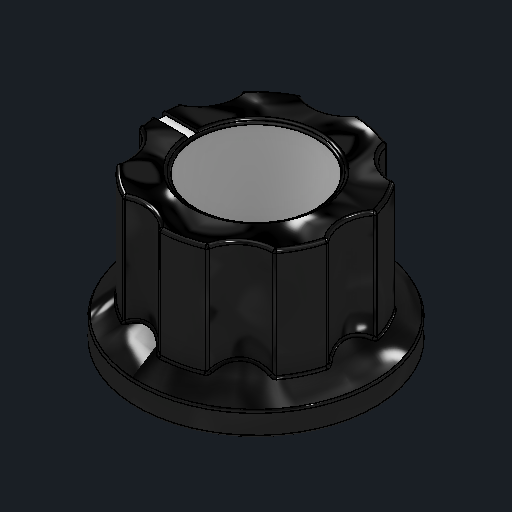
# Autodesk Inventor part: Knob2
Saved by Autodesk Inventor 2026.2 (Build 302298000, 298)
## iProperties
Created: 2015-05-06
Part Number: Knob2
Material: Generic
Document SubType Name: Modeling
Designer: Philip
Density: 1 g/cm^3
Appearance: Black
Author: Philip
Autodesk Inventor part; units mm, degrees
ref_plane "XZ Plane" through (0, 0, 0) normal (0, 1, 0) x (-1, 0, 0)
ref_plane "XY Plane" through (0, 0, 0) normal (0, 0, 1) x (1, 0, 0)
sketch "Sketch2" plane through (0, 0, 0) normal (0, 1, 0) x (-1, 0, 0)
  circle A0 centre (0, 0) radius 7.9375
  dimension "d0" = 15.875
  constraints: 1 centre point, 1 coincident
  measures "d0" diameter of A0
extrude "Extrusion1" add sketch "Sketch2" along normal blind 11.938
sketch "Sketch3" plane through (0, 11.938, 0) normal (0, 1, 0) x (1, 0, 0)
  circle A0 centre (0, 0) radius 7.9375 projected
  arc A1 (7.7055, 1.905) -> (7.7055, -1.905) centre (9.9648, 0) ccw
  line L0 (7.7055, -1.905) -> (7.7055, 1.905)
  dimension "d3" = 3.81
  constraints: 4 point on circle, 2 end point, 1 centre point, 1 vertical
  measures "d3" distance of L0.start L0.end
extrude "Extrusion2" cut sketch "Sketch3" against normal blind 11.938 contours A0 L0 | L0 A1
pattern_circular "Circular Pattern1" count 7 over 360 about axis through (0, 0, 0) along (0, 1, 0) of "Extrusion2"
sketch "Sketch4" plane through (0, 11.938, 0) normal (0, 1, 0) x (1, 0, 0)
  circle A0 centre (0, 0) radius 5.08
  dimension "d9" = 10.16
  constraints: 1 centre point, 1 coincident
  measures "d9" diameter of A0
extrude "Extrusion3" cut sketch "Sketch4" against normal blind 0.254
sketch "Sketch5" plane through (0, 0, 0) normal (1, 0, 0) x (0, 1, 0)
  line L0 (0, 0) -> (0, -9.525)
  line L1 (0, -9.525) -> (1.905, -9.525)
  line L2 (1.905, -9.525) -> (6.2153, -3.6691)
  line L3 (6.2153, -3.6691) -> (0, 0)
  line L4 (-2.3876, 0) -> (14.3256, 0) projected
  dimension "d12" = 9.525
  dimension "d13" = 1.905
  constraints: 8 end point, 1 perpendicular, 1 vertical
  measures "d12" distance of L0.start L0.end
  measures "d13" distance of L0.end L1.end
revolve "Revolution1" add sketch "Sketch5" angle 360 about axis through (0, -10, 0) along (0, 1, 0)
fillet "Fillet1" radius 0.254 31 edges at (0, 0, 9.525) (0, 1.905, 9.525) (-1.5598, 11.938, -6.8338) (0.1426, 7.5057, -7.9362) (-3.5719, 7.5057, -7.0884) (-6.1159, 7.5057, -5.0596) (-4.949, 11.938, -6.2058) (-6.3154, 11.938, -3.0413) (-7.769, 7.5057, -1.6269) (-7.769, 7.5057, 1.6269) (-7.9375, 11.938, 0) (-6.3154, 11.938, 3.0413) (-6.1159, 7.5057, 5.0596) (-3.5719, 7.5057, 7.0884) (-4.949, 11.938, 6.2058) (-1.5598, 11.938, 6.8338) (0.1426, 7.5057, 7.9362) (3.3149, 7.5057, 7.2122) (1.7663, 11.938, 7.7385) (4.3704, 11.938, 5.4803) (6.2937, 7.5057, 4.8367) (7.7055, 7.5057, 1.905) (7.1514, 11.938, 3.444) (7.0096, 11.938, 0) (7.7055, 7.5057, -1.905) (6.2937, 7.5057, -4.8367) (7.1514, 11.938, -3.444) (4.3704, 11.938, -5.4803) (3.3149, 7.5057, -7.2122) (1.7663, 11.938, -7.7385) (-5.08, 11.938, 0)
fillet "Fillet1" radius 0.254 16 edges at (-1.7312, 3.7511, -6.8) (-4.949, 3.0735, -6.2058) (-6.3154, 3.7565, -3.0414) (-7.9375, 3.0735, 0) (-6.3154, 3.7565, 3.0413) (-4.949, 3.0735, 6.2058) (-1.5598, 3.7565, 6.8338) (1.7663, 3.0735, 7.7385) (4.3703, 3.7565, 5.4803) (7.1514, 3.0735, 3.444) (7.0096, 3.7565, 0.0001) (7.1514, 3.0735, -3.444) (4.3704, 3.7565, -5.4802) (1.7663, 3.0735, -7.7385) (0.0738, 3.1388, -7.8484) (-5.08, 11.684, 0)
sketch "Sketch6" plane through (0, 11.938, 0) normal (0, 1, 0) x (1, 0, 0)
  circle A0 centre (0, 0) radius 5.046 projected
  line L0 (-5.0264, 0.4445) -> (-8.0286, 0.4445)
  line L1 (-8.0286, -0.4445) -> (-5.0264, -0.4445)
  arc A1 (-7.896, 1.5195) -> (-7.896, -1.5195) centre (0, 0) ccw projected
  dimension "d17" = 0.889
  dimension "d18" = 0.4445
  constraints: 4 end point, 4 point on circle, 2 horizontal
  measures "d17" distance between parallel lines of L1 L0
  measures "d18" distance from line of point (0, 0) L0
extrude "Extrusion4" cut sketch "Sketch6" against normal blind 0.254 contours A0 L1 A1 L0
ref_plane "Work Plane1" through (-7.9375, 0, 0) normal (1, 0, 0) x (0, 1, 0)
sketch "Sketch7" plane through (-7.9375, 0, 0) normal (1, 0, 0) x (0, 1, 0)
  line L0 (11.684, -0.4445) -> (11.684, 0.4445) projected
  line L1 (11.684, -0.4445) -> (3.2019, -0.4445)
  line L2 (3.2019, 1.5) -> (3.2019, -1.5) projected
  line L3 (11.684, 0.4445) -> (3.2019, 0.4445)
  point P0 (0, 0)
  constraints: 4 end point, 2 point on line, 1 horizontal, 1 perpendicular
extrude "Extrusion5" cut sketch "Sketch7" along normal blind 0.254
equation "\"d18\" = 0.5 * d17"
body "Solid1"
